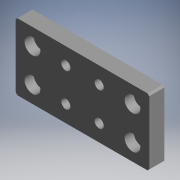
# Autodesk Inventor part: HBLPL5-4040
Saved by Autodesk Inventor 2017.3 (Build 213256000, 256)
## iProperties
Part Number: HBLPL5-4040
Material: Generic
Catalog Web Link: www.cadenas.de
Description: HBLPL-Plate Brackets
Vendor: MISUMI
Document SubType Name: Modeling
Designer: partserver
Manufacturer: MISUMI
Mass: 24.998 g
Surface Area: 99.5177 cm^2
Volume: 24.998 cm^3
Density: 1 g/cm^3
Appearance: PSOLRGB-175-175-175
Category: PARTsolutions
Company: MISUMI
Title: HBLPL5-4040
Author: Cadenas PARTsolutions
Comments: Plate Brackets
PSOL_IDENT_0: {$CADENAS_DATA\23d-libs\misumi\metric\38_al_extrusions_blackets\hblpl.prj},171 {VTYP=3D},{NB=HBLPL5-
PSOL_IDENT_1: 4040},{LINA=HBLPL5-4040},{NN=HBLPL},{DATE=08.06.2021 08:27:27},{GEOMDATE=31.03.2010 04:13:00},{VERSI
PSOL_IDENT_2: ON=},{LINEID=430},{WBVAR=ALT1,DC},{WBNUMERIC=DC}  {NB=HBLPL5-4040},{LINA=HBLPL5-4040},{KT=5},{PN=HBL
PSOL_IDENT_3: PL5-4040},{TPS=5-4040},{NO=5},{FRM=4040},{MAT=JIS SS400},{ST=Electroless Nickel Plating},{ALT1=},{DC=
PSOL_IDENT_4: 0},{A=80},{B=40},{T=9},{Z1=M5},{Z2=M5},{G=20},{E=10},{F=10.0},{MASS=0.21},{DD=5.500},{DD1=9.5},{HH=5
PSOL_IDENT_5: .500},{D=5.500},{D1=9.500},{H=5.500},{DCALG=[0]},{DCNB=}
NB: HBLPL5-4040
NN: HBLPL
NT: Plate Brackets
NBSYN: $PN.
LINA: HBLPL5-4040
CATALOG: Misumi
PN: HBLPL5-4040
TPS: 5-4040
NO: 5
FRM: 4040
MAT: JIS SS400
ST: Electroless Nickel Plating
ALT1: w/o DC (Through Hole)
DC: 0
A: 80
B: 40
T: 9
Z1: M5
Z2: M5
G: 20
E: 10
F: 10
MASS: 0.21
SUPPLIER: MISUMI
ARTICLENO: HBLPL5-4040
BOMINFO: HBLPL5-4040
CREATOR: CADENAS GmbH
Autodesk Inventor part; units mm, degrees
sketch "Sketch_4" plane through (0, 0, 0) normal (0, 1, 0) x (-1, 0, 0)
  line L0 (40, -19) -> (40, 19)
  line L1 (40, 19) -> (39, 20)
  line L2 (39, 20) -> (-39, 20)
  line L3 (-39, 20) -> (-40, 19)
  line L4 (-40, 19) -> (-40, -19)
  line L5 (-40, -19) -> (-39, -20)
  line L6 (-39, -20) -> (39, -20)
  line L7 (39, -20) -> (40, -19)
  constraints: 16 end point
extrude "Extrusion1" add sketch "Sketch_4" along normal blind 9
sketch "Sketch2" plane through (0, 0, 0) normal (0, -1, 0) x (1, 0, 0)
  point P0 (-30, 10)
hole "Hole1" at (-30, 0, 10) direction (0, 1, 0) diameter 5.5 depth 9 counterbore diameter 9.5 counterbore depth 5.5
pattern_linear "Rectangular Pattern1" count 2 spacing 60 along (1, 0, 0) count 2 spacing 20 along (0, 0, -1) of "Hole1"
sketch "Sketch3" plane through (0, 9, 0) normal (0, 1, 0) x (1, 0, 0)
  point P0 (-10, -10)
hole "Hole2" at (-10, 9, 10) direction (0, -1, 0) diameter 5.5 depth 9 counterbore diameter 9.5 counterbore depth 5.5
pattern_linear "Rectangular Pattern2" count 2 spacing 20 along (1, 0, 0) count 2 spacing 20 along (0, 0, -1) of "Hole2"
ref_plane "bolt4_1_XY" through (-10, 3.5, 10) normal (0, 1, 0) x (1, 0, 0)
ref_plane "bolt4_1_YZ" through (-10, 3.5, 10) normal (1, 0, 0) x (0, 0, -1)
ref_plane "bolt4_1_ZX" through (-10, 3.5, 10) normal (0, 0, -1) x (0, 1, 0)
ref_plane "bolt4_2_XY" through (10, 3.5, 10) normal (0, 1, 0) x (1, 0, 0)
ref_plane "bolt4_2_YZ" through (10, 3.5, 10) normal (1, 0, 0) x (0, 0, -1)
ref_plane "bolt4_2_ZX" through (10, 3.5, 10) normal (0, 0, -1) x (0, 1, 0)
ref_plane "bolt4_3_XY" through (-10, 3.5, -10) normal (0, 1, 0) x (1, 0, 0)
ref_plane "bolt4_3_YZ" through (-10, 3.5, -10) normal (1, 0, 0) x (0, 0, -1)
ref_plane "bolt4_3_ZX" through (-10, 3.5, -10) normal (0, 0, -1) x (0, 1, 0)
ref_plane "bolt4_4_XY" through (10, 3.5, -10) normal (0, 1, 0) x (1, 0, 0)
ref_plane "bolt4_4_YZ" through (10, 3.5, -10) normal (1, 0, 0) x (0, 0, -1)
ref_plane "bolt4_4_ZX" through (10, 3.5, -10) normal (0, 0, -1) x (0, 1, 0)
ref_plane "bolt5_1_XY" through (-30, 5.5, 10) normal (0, 1, 0) x (1, 0, 0)
ref_plane "bolt5_1_YZ" through (-30, 5.5, 10) normal (1, 0, 0) x (0, 0, -1)
ref_plane "bolt5_1_ZX" through (-30, 5.5, 10) normal (0, 0, -1) x (0, 1, 0)
ref_plane "bolt5_2_XY" through (30, 5.5, 10) normal (0, 1, 0) x (1, 0, 0)
ref_plane "bolt5_2_YZ" through (30, 5.5, 10) normal (1, 0, 0) x (0, 0, -1)
ref_plane "bolt5_2_ZX" through (30, 5.5, 10) normal (0, 0, -1) x (0, 1, 0)
ref_plane "bolt5_3_XY" through (-30, 5.5, -10) normal (0, 1, 0) x (1, 0, 0)
ref_plane "bolt5_3_YZ" through (-30, 5.5, -10) normal (1, 0, 0) x (0, 0, -1)
ref_plane "bolt5_3_ZX" through (-30, 5.5, -10) normal (0, 0, -1) x (0, 1, 0)
ref_plane "bolt5_4_XY" through (30, 5.5, -10) normal (0, 1, 0) x (1, 0, 0)
ref_plane "bolt5_4_YZ" through (30, 5.5, -10) normal (1, 0, 0) x (0, 0, -1)
ref_plane "bolt5_4_ZX" through (30, 5.5, -10) normal (0, 0, -1) x (0, 1, 0)
ref_plane "bracket_XY" through (0, 9, 0) normal (0, 1, 0) x (1, 0, 0)
ref_plane "bracket_YZ" through (0, 9, 0) normal (1, 0, 0) x (0, 0, -1)
ref_plane "bracket_ZX" through (0, 9, 0) normal (0, 0, -1) x (0, 1, 0)
body "Solid1"
